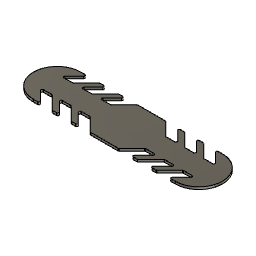
Mask holder (Autodesk Fusion 360 design; units mm, degrees)
Autodesk Fusion 360 part; units mm, degrees
sketch "Sketch1" plane through (0, 0, 0) normal (0, 0, 1) x (1, 0, 0) in component "mask holder"
  arc A0 (60, 0) -> (60, 20) centre (60, 10) ccw
  arc A1 (0, 20) -> (0, 0) centre (0, 10) ccw
  line L0 (30, -5.2068) -> (30, 28.719) construction
  line L1 (74.7629, 10) -> (-18.5863, 10) construction
  line L2 (60, 20) -> (57, 20)
  line L3 (57, 20) -> (62.6569, 14.3431)
  line L4 (57, 20) -> (62, 20) construction
  line L5 (62.6569, 14.3431) -> (57.6569, 14.3431)
  line L6 (57.6569, 14.3431) -> (52, 20)
  line L7 (52, 20) -> (49, 20)
  line L8 (49, 20) -> (54.6569, 14.3431)
  line L9 (44, 20) -> (41, 20)
  line L10 (54.6569, 14.3431) -> (49.6569, 14.3431)
  line L11 (41, 20) -> (46.6569, 14.3431)
  line L12 (49.6569, 14.3431) -> (44, 20)
  line L13 (46.6569, 14.3431) -> (41.6569, 14.3431)
  line L14 (41.6569, 14.3431) -> (36, 20)
  line L15 (11, 20) -> (5.3431, 14.3431)
  line L16 (19, 20) -> (13.3431, 14.3431)
  line L17 (3, 20) -> (-2, 20) construction
  line L18 (3, 20) -> (-2.6569, 14.3431)
  line L19 (0, 20) -> (3, 20)
  line L20 (5.3431, 14.3431) -> (10.3431, 14.3431)
  line L21 (-2.6569, 14.3431) -> (2.3431, 14.3431)
  line L22 (2.3431, 14.3431) -> (8, 20)
  line L23 (18.3431, 14.3431) -> (24, 20)
  line L24 (13.3431, 14.3431) -> (18.3431, 14.3431)
  line L25 (10.3431, 14.3431) -> (16, 20)
  line L26 (16, 20) -> (19, 20)
  line L27 (8, 20) -> (11, 20)
  line L28 (24, 20) -> (36, 20)
  line L29 (11, 0) -> (5.3431, 5.6569)
  line L30 (41, 0) -> (46.6569, 5.6569)
  line L31 (30, 25.2068) -> (30, -8.719) construction
  line L32 (13.3431, 5.6569) -> (18.3431, 5.6569)
  line L33 (46.6569, 5.6569) -> (41.6569, 5.6569)
  line L34 (5.3431, 5.6569) -> (10.3431, 5.6569)
  line L35 (16, 0) -> (19, 0)
  line L36 (3, 0) -> (-2, 0) construction
  line L37 (3, 0) -> (-2.6569, 5.6569)
  line L38 (10.3431, 5.6569) -> (16, 0)
  line L39 (54.6569, 5.6569) -> (49.6569, 5.6569)
  line L40 (0, 0) -> (3, 0)
  line L41 (19, 0) -> (13.3431, 5.6569)
  line L42 (49.6569, 5.6569) -> (44, 0)
  line L43 (57.6569, 5.6569) -> (52, 0)
  line L44 (49, 0) -> (54.6569, 5.6569)
  line L45 (24, 0) -> (36, 0)
  line L46 (44, 0) -> (41, 0)
  line L47 (18.3431, 5.6569) -> (24, 0)
  line L48 (41.6569, 5.6569) -> (36, 0)
  line L49 (8, 0) -> (11, 0)
  line L50 (57, 0) -> (62, 0) construction
  line L51 (62.6569, 5.6569) -> (57.6569, 5.6569)
  line L52 (60, 0) -> (57, 0)
  line L53 (57, 0) -> (62.6569, 5.6569)
  line L54 (-2.6569, 5.6569) -> (2.3431, 5.6569)
  line L55 (2.3431, 5.6569) -> (8, 0)
  line L56 (52, 0) -> (49, 0)
  point P0 (0, 10)
  point P1 (60, 10)
  point P2 (0, 10)
  point P3 (0, 10)
  dimension "d5" = 20
  dimension "d6" = 60
  dimension "d7" = 3
  dimension "d8" = 8
  dimension "d9" = 45
  dimension "d12" = 5
  dimension "d15" = 8
  dimension "d16" = 3
  dimension "d17" = 8
  dimension "d19" = 5
  dimension "d20" = 8
  dimension "d21" = 3
  dimension "d22" = 8
  dimension "d23" = 5
  dimension "d24" = 8
  constraint perpendicular L0 L1
  constraint horizontal L2
  constraint horizontal L4
  constraint parallel L1 L5
  constraint parallel L3 L6
  constraint parallel L2 L7
  constraint parallel L6 L8
  constraint parallel L11 L12
  constraint horizontal L13
  constraint parallel L11 L14
  constraint symmetric A0.end L0 A1.start
  constraint symmetric P1 L0 P3
  constraint symmetric L0 L2.end L17.start
  constraint symmetric L0 L3.end L18.end
  constraint symmetric L0 L4.end L17.end
  constraint symmetric L0 L5.end L21.end
  constraint symmetric L0 L6.end L22.end
  constraint symmetric L0 L7.end L15.start
  constraint symmetric L0 L8.end L15.end
  constraint symmetric L0 L9.start L25.end
  constraint symmetric L0 L9.end L16.start
  constraint symmetric L0 L10.end L20.end
  constraint symmetric L0 L11.end L16.end
  constraint symmetric L0 L13.end L23.start
  constraint symmetric L0 L14.end L23.end
  constraint symmetric A0.end L1 A0.start
  constraint symmetric A1.start L1 A1.end
  constraint symmetric P3 L1 P2
  constraint symmetric P1 L1 A0.centre
  constraint symmetric L0.start L1 L31.start
  constraint symmetric L0.end L1 L31.end
  constraint symmetric L1 L2.end L50.start
  constraint symmetric L1 L3.end L51.start
  constraint symmetric L1 L4.end L50.end
  constraint symmetric L1 L5.end L43.start
  constraint symmetric L1 L6.end L43.end
  constraint symmetric L1 L7.end L44.start
  constraint symmetric L1 L8.end L39.start
  constraint symmetric L1 L9.start L42.end
  constraint symmetric L1 L9.end L30.start
  constraint symmetric L1 L10.end L39.end
  constraint symmetric L1 L11.end L30.end
  constraint symmetric L1 L13.end L33.end
  constraint symmetric L1 L14.end L45.end
  constraint symmetric L1 L23.start L32.end
  constraint symmetric L1 A1.start A1.end
  constraint symmetric L1 L17.end L36.end
  constraint symmetric L1 L23.end L45.start
  constraint symmetric L1 L15.end L29.end
  constraint symmetric L1 L16.end L32.start
  constraint symmetric L1 L15.start L29.start
  constraint symmetric L1 P3 P2
  constraint symmetric L1 L22.end L49.start
  constraint symmetric L1 L21.end L54.end
  constraint symmetric L1 L20.end L34.end
  constraint symmetric L1 L16.start L35.end
  constraint symmetric L1 L25.end L35.start
  constraint symmetric L1 L17.start L36.start
  constraint symmetric L1 L18.end L37.end
  measures "d5" distance of A1.end A1.start
  measures "d6" distance of A1.end A0.start
  measures "d7" distance of A0.end L2.end
  measures "d8" distance of L2.end L3.end
  measures "d9" angle of L3 L4
  measures "d12" distance of L3.end L5.end
  measures "d15" distance of L5.end L6.end
  measures "d16" distance of L6.end L7.end
  measures "d17" distance of L7.end L8.end
  measures "d19" distance of L8.end L10.end
  measures "d20" distance of L9.start L10.end
  measures "d21" distance of L9.start L9.end
  measures "d22" distance of L9.end L11.end
  measures "d23" distance of L11.end L13.end
  measures "d24" distance of L13.end L14.end
extrude "Extrude1" add sketch "Sketch1" along normal blind 1
fillet "Fillet1" radius 0.5 46 edges at (57, 0, 0.5) (62.6569, 5.6569, 0.5) (57.6569, 5.6569, 0.5) (52, 0, 0.5) (49, 0, 0.5) (54.6569, 5.6569, 0.5) (46.6569, 5.6569, 0.5) (41, 0, 0.5) (36, 0, 0.5) (41.6569, 5.6569, 0.5) (18.3431, 5.6569, 0.5) (24, 0, 0.5) (13.3431, 5.6569, 0.5) (19, 0, 0.5) (16, 0, 0.5) (5.3431, 5.6569, 0.5) (11, 0, 0.5) (8, 0, 0.5) (3, 0, 0.5) (-2.6569, 5.6569, 0.5) (10.3431, 5.6569, 0.5) (2.3431, 5.6569, 0.5) (2.3431, 14.3431, 0.5) (3, 20, 0.5) (8, 20, 0.5) (10.3431, 14.3431, 0.5) (16, 20, 0.5) (19, 20, 0.5) (18.3431, 14.3431, 0.5) (24, 20, 0.5) (13.3431, 14.3431, 0.5) (5.3431, 14.3431, 0.5) (11, 20, 0.5) (-2.6569, 14.3431, 0.5) (36, 20, 0.5) (41.6569, 14.3431, 0.5) (46.6569, 14.3431, 0.5) (41, 20, 0.5) (44, 20, 0.5) (49.6569, 14.3431, 0.5) (54.6569, 14.3431, 0.5) (49, 20, 0.5) (52, 20, 0.5) (57.6569, 14.3431, 0.5) (62.6569, 14.3431, 0.5) (57, 20, 0.5)
component "mask holder" placed x (1, 0, 0) y (0, 1, 0) z (0, 0, 1) at (0, 0, 0)
equation "length = 80 mm"
equation "width = 20 mm"
equation "thickness = 1 mm"
equation "finalLength = length - width"
equation "d5 = width"
equation "d6 = finalLength"
equation "d7 = L3"
equation "d8 = L"
equation "L = 8 mm"
equation "L2 = 5 mm"
equation "d12 = L2"
equation "L3 = 3 mm"
equation "d15 = L"
equation "d16 = L3"
equation "d17 = L"
equation "d19 = L2"
equation "d20 = L"
equation "d21 = L3"
equation "d22 = L"
equation "d23 = L2"
equation "d24 = L"
